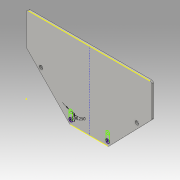
# Autodesk Inventor part: new pulley plate
Saved by Autodesk Inventor 2016 (Build 200138000, 138)
## iProperties
Created: 2015-11-24
Part Number: new pulley plate
Material: Generic
Document SubType Name: Modeling
Designer: Delta
Density: 1 g/cm^3
Appearance: Default
Author: Delta
Autodesk Inventor part; units mm, degrees
note: some values were not read from the file. Chosen so that the rebuilt part matches the saved one: sketch regions of "Extrusion2".
ref_plane "YZ Plane" through (0, 0, 0) normal (1, 0, 0) x (0, 1, 0)
ref_plane "XZ Plane" through (0, 0, 0) normal (0, 1, 0) x (-1, 0, 0)
ref_plane "XY Plane" through (0, 0, 0) normal (0, 0, 1) x (1, 0, 0)
sketch "Sketch1" plane through (0, 0, 0) normal (0, 0, 1) x (1, 0, 0)
  line L0 (0, 0) -> (215.9, 0)
  line L1 (215.9, 0) -> (215.9, 152.4)
  line L2 (215.9, 152.4) -> (0, 152.4)
  line L3 (0, 152.4) -> (0, 0)
  dimension "d0" = 215.9
  dimension "d1" = 152.4
  constraints: 8 end point, 2 parallel, 1 horizontal, 1 perpendicular
  measures "d0" distance of L2.end L1.end
  measures "d1" distance of L1.end L0.end
extrude "Extrusion1" add sketch "Sketch1" along normal blind 3.175
sketch "Sketch2" plane through (0, 0, 3.175) normal (0, 0, 1) x (1, 0, 0)
  line L0 (215.9, 152.4) -> (0, 152.4) construction
  line L1 (107.95, 152.4) -> (107.95, 0) construction
  line L2 (0, 0) -> (215.9, 0) projected
  point P0 (25.4, 59.8875)
  point P1 (76.2, 7.5)
  point P2 (190.5, 59.8875)
  point P3 (139.7, 7.5)
  dimension "d5" = 31.75
  dimension "d7" = 82.55
  dimension "d9" = 52.3875
  dimension "d10" = 7.5
  constraints: 2 end point, 2 symmetric about line, 1 midpoint, 1 vertical
  measures "d5" distance from line of L1 point (76.2, 7.5)
  measures "d7" distance from line of L1 point (25.4, 59.888)
  measures "d9" vertical distance of point (25.4, 59.888) point (76.2, 7.5)
  measures "d10" distance from line of L2 point (76.2, 7.5)
hole "Hole1" at (25.4, 59.8875, 3.175) at (76.2, 7.5, 3.175) at (190.5, 59.8875, 3.175) at (139.7, 7.5, 3.175) direction (0, 0, -1) diameter 6.35 end through all
sketch "Sketch3" plane through (0, 0, 3.175) normal (0, 0, 1) x (1, 0, 0)
  line L0 (215.9, 152.4) -> (0, 152.4) projected
  line L1 (107.95, 152.4) -> (107.95, 0)
  line L2 (0, 0) -> (215.9, 0) projected
  circle A0 centre (25.4, 59.8875) radius 3.175 projected
  circle A1 centre (76.2, 7.5) radius 3.175 projected
  line L3 (25.4, 59.8875) -> (76.2, 7.5) construction
  line L4 (0.8957, 76.0359) -> (73.692, 0.9647)
  line L5 (0, 152.4) -> (0, 0) projected
  line L6 (0, 130.175) -> (0, 78.2462)
  line L7 (3.175, 133.35) -> (107.95, 133.35)
  line L8 (0, 133.35) -> (0, 125.3708)
  circle A2 centre (190.5, 59.8875) radius 3.175
  circle A3 centre (139.7, 7.5) radius 3.175
  line L9 (190.5, 59.8875) -> (139.7, 7.5) construction
  line L10 (215.0043, 76.0359) -> (142.208, 0.9647)
  line L11 (215.9, 152.4) -> (215.9, 78.2462)
  line L12 (215.9, 133.35) -> (215.9, 76.9596)
  line L13 (212.725, 133.35) -> (107.95, 133.35)
  line L14 (215.9, 130.175) -> (215.9, 125.3708)
  arc A4 (3.175, 133.35) -> (0, 130.175) centre (3.175, 130.175) ccw
  arc A5 (0, 78.2462) -> (0.8957, 76.0359) centre (3.175, 78.2462) ccw
  line L15 (75.9713, 0) -> (107.95, 0)
  line L16 (139.9287, 0) -> (107.95, 0)
  arc A6 (73.692, 0.9647) -> (75.9713, 0) centre (75.9713, 3.175) ccw
  arc A7 (139.9287, 0) -> (142.208, 0.9647) centre (139.9287, 3.175) ccw
  arc A8 (215.0043, 76.0359) -> (215.9, 78.2462) centre (212.725, 78.2462) ccw
  arc A9 (215.9, 130.175) -> (212.725, 133.35) centre (212.725, 130.175) ccw
  line L17 (215.9, 0) -> (215.9, 152.4) projected
  point P0 (74.6275, 0)
  point P1 (0, 76.9596)
  point P2 (77.9849, 0)
  dimension "d19" = 6.35
  dimension "d20" = 19.05
  dimension "d21" = 3.175
  dimension "d22" = 3.175
  dimension "d23" = 3.175
  dimension "d27" = 31.9787
  dimension "d28" = 31.9787
  constraints: 28 end point, 19 point on line, 12 point on circle, 12 tangent, 8 centre point, 5 symmetric about line, 3 collinear, 3 equal radius, 2 midpoint, 1 parallel, 1 perpendicular, 1 vertical, 2 other
  measures "d19" distance between parallel lines of L3 L4
  measures "d20" distance between parallel lines of L7 L0
  measures "d21" radius of A4
  measures "d22" radius of A6
  measures "d23" radius of A8
  measures "d27" distance from line of L1 A6.centre
  measures "d28" distance from line of A7.centre L1
extrude "Extrusion2" cut sketch "Sketch3" against normal blind 3.175 contours L11 A9 L13 L1 L0 | L1 L7 A4 L5 L0 | L2 L5 A5 L4 A6 | A7 L10 A8 L12 L17 L2
sketch "Sketch4" plane through (0, 0, 3.175) normal (0, 0, 1) x (1, 0, 0)
  circle A0 centre (76.2059, 20.2) radius 3.175
  circle A1 centre (76.2, 7.5) radius 3.175 projected
  line L0 (73.0309, 20.2015) -> (73.0254, 7.4505)
  circle A2 centre (76.2, 7.5) radius 3.175 projected
  line L1 (79.3809, 20.2) -> (79.375, 7.4971)
  line L2 (3.175, 133.35) -> (212.725, 133.35) projected
  line L3 (107.95, 133.35) -> (107.95, 0) construction
  line L4 (75.9713, 0) -> (139.9287, 0) projected
  circle A3 centre (139.6941, 20.2) radius 3.175
  line L5 (142.8691, 20.2015) -> (142.8746, 7.4505)
  line L6 (136.5191, 20.2) -> (136.525, 7.5)
  circle A4 centre (76.2, 7.5) radius 3.175
  circle A5 centre (139.7, 7.5) radius 3.175 projected
  circle A6 centre (139.7, 7.5) radius 3.175
  point P0 (0, 0)
  point P1 (136.525, 7.4971)
  dimension "d29" = 6.35
  dimension "d30" = 12.7
  constraints: 11 point on circle, 10 end point, 5 symmetric about line, 3 centre point, 2 coincident, 2 midpoint, 2 point on line, 4 other
  measures "d29" diameter of A0
  measures "d30" distance of A1.centre A0.centre
equation "\"d28\" = d27"
body "Solid1"
